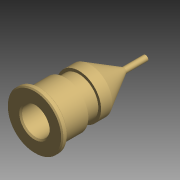
# Autodesk Inventor part: Nozzle
Saved by Autodesk Inventor 2015 (Build 190159000, 159)
## iProperties
Created: 2015-01-06
Part Number: Nozzle
Material: Generic
Document SubType Name: Modeling
Designer: ice
Density: 1 g/cm^3
Appearance: Default
Mass: 0.47413 g
Surface Area: 6.40818 cm^2
Volume: 0.47413 cm^3
Author: ice
Autodesk Inventor part; units mm, degrees
ref_plane "YZ Plane" through (0, 0, 0) normal (1, 0, 0) x (0, 1, 0)
ref_plane "XZ Plane" through (0, 0, 0) normal (0, 1, 0) x (-1, 0, 0)
sketch "Sketch1" plane through (0, 0, 0) normal (0, 0, 1) x (1, 0, 0)
  line L0 (0, 14.375) -> (0, 5.6)
  line L1 (0, 14.375) -> (0, 17.5)
  line L2 (0, 17.5) -> (0, 5.6)
  line L3 (-0.35, 17.5) -> (0, 17.5)
  line L4 (-5, 7.5) -> (6.0041, 7.5) construction
  line L5 (-5, -2.5) -> (-2.8, -2.5)
  line L6 (-2.8, -2.5) -> (0, -2.5)
  line L7 (0, -2.5) -> (0, 5.6)
  line L8 (0, -2.5) -> (-2.5, -2.5)
  line L9 (0, -2.5) -> (-4, -2.5)
  line L10 (0, -2.5) -> (-4, -2.5)
  line L11 (-3.5, 3) -> (-3.5, 5.5)
  line L12 (-3.5, 5.5) -> (-4, 5.5)
  line L13 (-4, 5.5) -> (-4, 7.5)
  line L14 (-5, -2.5) -> (-5, -1.5)
  line L15 (-5, -1.5) -> (-4, -1.5)
  line L16 (-4, 7.5) -> (5.0041, 7.5) construction
  line L17 (-4, 7.5) -> (-0.5, 13.5622)
  line L18 (0, 17.5) -> (-0.5, 17.5)
  line L19 (-0.5, 17.5) -> (-0.5, 13.5622)
  line L20 (-4, 7.5) -> (-2.8, 7.5)
  line L21 (-4, -1.5) -> (-4.2, -1.5)
  line L22 (-4.2, -1.5) -> (-4.2, 3)
  line L23 (-4.2, 3) -> (-3.5, 3)
  dimension "d82" = 10
  dimension "d106" = 20
  dimension "d107" = 5
  dimension "d150" = 2.5
  dimension "d151" = 0.5
  dimension "d153" = 90
  dimension "d154" = 1
  dimension "d157" = 1
  dimension "d159" = 2
  dimension "d161" = 0.5
  dimension "d162" = 6.0622
  dimension "d163" = 3.9378
  dimension "d164" = 60
  dimension "d175" = 4
  dimension "d176" = 0.2
  constraints: 48 end point, 5 point on line, 4 horizontal, 4 perpendicular, 2 collinear, 2 vertical
  measures "d82" vertical distance of L3.start L4.start
  measures "d106" distance of L1.end L6.end
  measures "d107" distance of L6.end L5.start
  measures "d150" distance of L11.start L11.end
  measures "d151" distance of L11.end L12.end
  measures "d153" angle of L12 L13
  measures "d154" distance of L5.start L14.end
  measures "d157" distance of L15.end L14.end
  measures "d159" distance of L13.end L12.end
  measures "d161" distance of L1.end L18.end
  measures "d162" vertical distance of L13.end L17.end
  measures "d163" distance of L18.end L17.end
  measures "d164" angle of L17 L4
  measures "d175" distance from line of L7 L15.end
  measures "d176" distance of L15.end L21.end
revolve "Revolution1" add sketch "Sketch1" angle 360 about axis through (0, 14.375, 0) along (0, -1, 0)
ref_plane "Work Plane3" through (0, -2.5, 0) normal (0, 1, 0) x (-1, 0, 0)
sketch "Sketch5" plane through (0, -2.5, 0) normal (0, 1, 0) x (-1, 0, 0)
  point P0 (0, 0)
sketch "Sketch6" plane through (0, -2.5, 0) normal (0, -1, 0) x (1, 0, 0)
  circle A0 centre (0, 0) radius 2.9
  dimension "d108" = 5.8
  constraints: 1 centre point, 1 coincident
  measures "d108" diameter of A0
hole "Hole6" at (0, -2.5, 0) direction (0, 1, 0) diameter 5 depth 7.25 tip angle 118
hole "Hole7" at (0, -2.5, 0) direction (0, 1, 0) diameter 2 depth 13 tip angle 118
chamfer "Chamfer1" distance 0.25 angle 45 1 edges at (0, -2.5, 2.5)
sketch "Sketch8" plane through (0, 17.5, 0) normal (0, 1, 0) x (1, 0, 0)
  point P0 (0, 0)
hole "Hole9" at (0, 17.5, 0) direction (0, -1, 0) diameter 0.25 end through all
chamfer "Chamfer2" distance 0.2 angle 45 2 edges at (5, -1.5, 0) (5, -2.5, 0)
body "Solid1"
